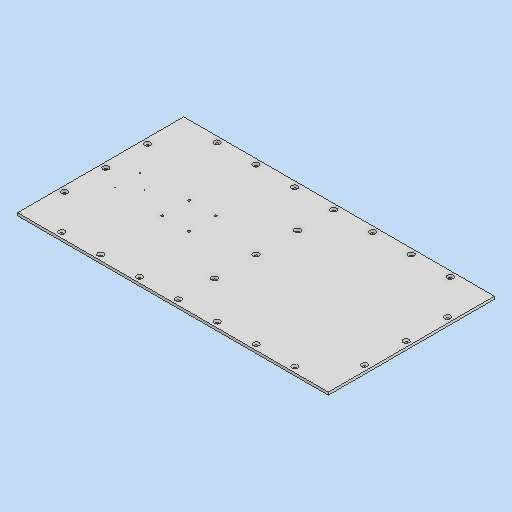
# Autodesk Inventor part: вверхняя плита
Saved by Autodesk Inventor 2025 (Build 290162000, 162)
## iProperties
Created: 2025-02-24
Part Number: вверхняя плита
Material: Типовые
Document SubType Name: Modeling
Designer: volko
Density: 1 g/cm^3
Appearance: По умолчанию
Author: volko
Autodesk Inventor part; units mm, degrees
ref_plane "YZ Plane" through (0, 0, 0) normal (1, 0, 0) x (0, 1, 0)
ref_plane "XZ Plane" through (0, 0, 0) normal (0, 1, 0) x (-1, 0, 0)
ref_plane "XY Plane" through (0, 0, 0) normal (0, 0, 1) x (1, 0, 0)
sketch "Эскиз1" plane through (0, 0, 0) normal (0, 1, 0) x (-1, 0, 0)
  line L0 (-290, 155) -> (-290, -155)
  line L1 (290, -155) -> (290, 155)
  line L2 (0, -217) -> (0, 217) projected
  line L3 (406, 0) -> (-406, 0) projected
  line L4 (290, 155) -> (-290, 155)
  line L5 (-125, 155) -> (-290, 155)
  line L6 (290, -155) -> (-290, -155)
  point P0 (0, 0)
  dimension "d0" = 580
  dimension "d1" = 310
  constraints: 10 end point, 3 horizontal, 2 perpendicular, 1 collinear, 1 parallel, 2 other
  measures "d0" distance of L0.start L1.end
  measures "d1" distance of L1.start L1.end
extrude "Выдавливание1" add sketch "Эскиз1" along normal blind 5
sketch "Эскиз2" plane through (0, 5, 0) normal (0, 1, 0) x (1, 0, 0)
  line L0 (0, 217) -> (0, -217) projected
  line L1 (-406, 0) -> (406, 0) projected
  line L2 (290, 155) -> (-290, 155) projected
  line L3 (290, -155) -> (290, 155) projected
  point P0 (0, 0)
  point P1 (0, 0)
  point P2 (280, 77.5)
  point P3 (0, 0)
  point P4 (280, 0)
  point P5 (280, -77.5)
  point P6 (0, 77.5)
  point P7 (0, 0)
  point P8 (0, -77.5)
  point P9 (-280, 77.5)
  point P10 (-280, 0)
  point P11 (-280, -77.5)
  point P12 (217.5, 145)
  point P13 (145, 145)
  point P14 (72.5, 145)
  point P15 (0, 145)
  point P16 (-72.5, 145)
  point P17 (-145, 145)
  point P18 (-217.5, 145)
  point P19 (217.5, -145)
  point P20 (145, -145)
  point P21 (72.5, -145)
  point P22 (0, -145)
  point P23 (-72.5, -145)
  point P24 (-145, -145)
  point P25 (-217.5, -145)
  dimension "d44" = 77.5
  dimension "d45" = 10
  dimension "d48" = 77.5
  dimension "d51" = 280
  dimension "d54" = 10
  dimension "d55" = 72.5
  dimension "d58" = 72.5
  dimension "d61" = 290
  constraints: 2 horizontal, 2 vertical, 1 coincident, 21 other
  measures "d44" distance from line of L2 point (280, 77.5)
  measures "d45" distance from line of L3 point (280, 77.5)
  measures "d48" distance of point (280, 77.5) point (280, 0)
  measures "d51" distance of point (280, 77.5) point (0, 77.5)
  measures "d54" distance from line of point (217.5, 145) L2
  measures "d55" distance from line of L3 point (217.5, 145)
  measures "d58" distance of point (217.5, 145) point (145, 145)
  measures "d61" distance of point (217.5, 145) point (217.5, -145)
hole "Отверстие1" at (-217.5, 5, 145) at (-145, 5, 145) at (-72.5, 5, 145) at (-217.5, 5, -145) at (-145, 5, -145) at (-72.5, 5, -145) at (-280, 5, 77.5) at (-280, 5, 0) at (-280, 5, -77.5) at (0, 5, 145) at (72.5, 5, 145) at (145, 5, 145) at (217.5, 5, 145) at (0, 5, -145) at (72.5, 5, -145) at (145, 5, -145) at (217.5, 5, -145) at (0, 5, 77.5) at (0, 5, 0) at (0, 5, -77.5) at (280, 5, 77.5) at (280, 5, 0) at (280, 5, -77.5) direction (0, -1, 0) diameter 5.5 end through all countersink diameter 11 countersink angle 90
sketch "Эскиз3" plane through (0, 5, 0) normal (0, 1, 0) x (1, 0, 0)
  line L0 (-406, 0) -> (406, 0) projected
  line L1 (0, 217) -> (0, -217) projected
  point P0 (0, 0)
  point P1 (-150, 25)
  point P2 (-100, 25)
  point P3 (-150, -25)
  point P4 (-100, -25)
  dimension "d73" = 50
  dimension "d76" = 50
  dimension "d79" = 100
  constraints: 1 horizontal, 1 symmetric about line, 1 vertical, 3 other
  measures "d73" distance of point (-150, 25) point (-100, 25)
  measures "d76" distance of point (-150, 25) point (-150, -25)
  measures "d79" distance from line of L1 point (-100, 25)
hole "Отверстие2" at (-150, 5, -25) at (-100, 5, 25) at (-100, 5, -25) at (-150, 5, 25) direction (0, -1, 0) diameter 4.134 end through all thread size "M5x0.8" class "6H" standard "ISO Metric profile"
sketch "Эскиз4" plane through (0, 5, 0) normal (0, 1, 0) x (1, 0, 0)
  line L0 (-406, 0) -> (406, 0) projected
  line L1 (-290, 155) -> (-290, -155) construction
  point P0 (0, 0)
  point P1 (-240, 23.4)
  point P2 (-240, -23.4)
  point P3 (-208.083, 0)
  dimension "d87" = 46.8
  dimension "d88" = 31.917
  dimension "d89" = 50
  constraints: 1 point on line, 1 symmetric about line
  measures "d87" distance of point (-240, -23.4) point (-240, 23.4)
  measures "d88" horizontal distance of point (-240, 23.4) point (-208.083, 0)
  measures "d89" distance from line of point (-240, 23.4) L1
hole "Отверстие3" at (-240, 5, -23.4) at (-208.083, 5, 0) at (-240, 5, 23.4) direction (0, -1, 0) diameter 1.567 end through all thread size "M2x0.4" class "6H" standard "ISO Metric profile"
